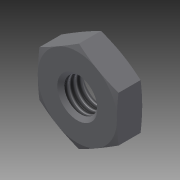
# Autodesk Inventor part: D-5288
Saved by Autodesk Inventor 2014 (Build 180170000, 170)
## iProperties
Category: PARTsolutions
Company: BIMBA
Created: 2014-01-19
Part Number: D-5288
Material: Generic
Catalog Web Link: www.cadenas.de
Description: Mounting Nut for Original Line Cylinders-
Vendor: BIMBA
Document SubType Name: Standard Catalog Part
Designer: Michael
Manufacturer: BIMBA
Density: 1 g/cm^3
Appearance: RGB(191.25000000000000,191.25000000000000,191.25000000000000)
PSOL_IDENT_0: {$CADENAS_DATA\23d-libs\bimba\bimba\bimba_imperial\bimba_full_line\original_line_cylinders\accessori
PSOL_IDENT_1: es\mounting_nut.prj},192 {VTYP=3D},{NB=D-5288},{LINA=D-5288},{NN=Mounting Nut for Original Line Cyli
PSOL_IDENT_2: nders},{DATE=11.06.2012 07:31:25},{GEOMDATE=10.11.2011 00:00:00},{VERSION=},{LINEID=210},{LINESUBID=
PSOL_IDENT_3: -1},{WBVAR=MAT}  {NB=D-5288},{LINA=D-5288},{KT=DUMMY},{PN=D-5288},{PN1=D-5288},{C=#10-32},{TH=UNF},{
PSOL_IDENT_4: MAT=},{MAT1='','Zinc-Plated Carbon Steel', '-SS', 'Stainless Steel'},{A=0.38},{A1=0.37500000},{B=0.1
PSOL_IDENT_5: 2},{B1=0.12000000},{NDM=0.19000000},{PITCH=0.0313},{DIA=-},{DIA2=-},{DIA3=-},{DIA1=0},{DIA4=0.000000
PSOL_IDENT_6: 00},{DIA5=0.00000000},{T=-},{T2=-},{T3=-},{T1=0},{T4=0.00000000},{T5=0.00000000},{COLOR=0.75,0.75,0.
PSOL_IDENT_7: 75,0.00},{TT=0.05000000},{TO=0.20000000},{PRA=1}
CNS_NN: Mounting Nut for Original Line Cylinders
CNS_NB: D-5288
CNS_NBSYN: $PN.
CNS_LINA: D-5288
CNS_PN: D-5288
CNS_PN1: D-5288
CNS_C: #10-32
CNS_TH: UNF
CNS_MAT: Zinc-Plated Carbon Steel
CNS_MAT1: '','Zinc-Plated Carbon Steel', '-SS', 'Stainless Steel'
CNS_A: 0.38
CNS_A1: 0.37500000
CNS_B: 0.12
CNS_B1: 0.12000000
CNS_NDM: 0.19000000
CNS_PITCH: 0.0313
CNS_DIA: -
CNS_DIA2: -
CNS_DIA3: -
CNS_DIA1: 0.000
CNS_DIA4: 0.00000000
CNS_DIA5: 0.00000000
CNS_T: -
CNS_T2: -
CNS_T3: -
CNS_T1: 0.000
CNS_T4: 0.00000000
CNS_T5: 0.00000000
CNS_COLOR: 0.75,0.75,0.75,0.00
CNS_TT: 0.05000000
CNS_TO: 0.20000000
CNS_PRA: 1
SUPPLIER: BIMBA
ARTICLENO: D-5288
BOMINFO: D-5288
CREATOR: CADENAS GmbH
Title: D-5288
Author: Cadenas PARTsolutions
Autodesk Inventor part; units mm, degrees
sketch "Sketch_8" plane through (0, 0, 0) normal (1, 0, 0) x (0, 1, 0)
  line L0 (0, -3.048) -> (0, 0)
  line L1 (0, 0) -> (4.7625, 0)
  line L2 (4.7625, 0) -> (5.715, -0.2552)
  line L3 (5.715, -0.2552) -> (5.715, -2.7928)
  line L4 (5.715, -2.7928) -> (4.7625, -3.048)
  line L5 (4.7625, -3.048) -> (0, -3.048)
  line L6 (0, -3.048) -> (0, 0)
  constraints: 14 end point
sketch "Sketch_10" plane through (0, 0, 0) normal (0, 0, 1) x (1, 0, 0)
  line L0 (-9.525, 9.525) -> (-9.525, -9.525)
  line L1 (-9.525, -9.525) -> (9.525, -9.525)
  line L2 (9.525, -9.525) -> (9.525, 9.525)
  line L3 (9.525, 9.525) -> (-9.525, 9.525)
  line L4 (-4.7625, 2.7496) -> (-4.7625, -2.7496)
  line L5 (-4.7625, -2.7496) -> (0, -5.4993)
  line L6 (0, -5.4993) -> (4.7625, -2.7496)
  line L7 (4.7625, -2.7496) -> (4.7625, 2.7496)
  line L8 (4.7625, 2.7496) -> (0, 5.4993)
  line L9 (0, 5.4993) -> (-4.7625, 2.7496)
  constraints: 20 end point
revolve "Revolution1" add sketch "Sketch_8" angle 360 about axis through (0, 0, -3.048) along (0, 0, -1)
extrude "Extrusion1" cut sketch "Sketch_10" against normal blind 3.048
sketch "Sketch_11" plane through (0, 0, 0) normal (1, 0, 0) x (0, 1, 0)
  line L0 (0, -3.048) -> (0, 0)
  line L1 (0, 0) -> (2.413, 0)
  line L2 (2.413, 0) -> (1.9837, -0.4293)
  line L3 (1.9837, -0.4293) -> (1.9837, -2.6187)
  line L4 (1.9837, -2.6187) -> (2.413, -3.048)
  line L5 (2.413, -3.048) -> (0, -3.048)
  line L6 (0, -3.048) -> (0, 0)
  constraints: 14 end point
revolve "Revolution2" cut sketch "Sketch_11" angle 360 about axis through (0, 0, -3.048) along (0, 0, -1)
thread "Thread1" size "10-32 UNF" class "2B" standard "ANSI Unified Screw Threads" full length
ref_plane "NUT_XY" through (0, 0, 0) normal (0, 0, 1) x (1, 0, 0)
ref_plane "NUT_YZ" through (0, 0, 0) normal (1, 0, 0) x (0, 1, 0)
ref_plane "NUT_ZX" through (0, 0, 0) normal (0, 1, 0) x (0, 0, 1)
ref_plane "a1_XY" through (-4.7625, 4.7625, 0) normal (0, 0, 1) x (1, 0, 0)
ref_plane "a1_YZ" through (-4.7625, 4.7625, 0) normal (1, 0, 0) x (0, 1, 0)
ref_plane "a1_ZX" through (-4.7625, 4.7625, 0) normal (0, 1, 0) x (0, 0, 1)
ref_plane "a2_XY" through (4.7625, 4.7625, 0) normal (0, 0, 1) x (1, 0, 0)
ref_plane "a2_YZ" through (4.7625, 4.7625, 0) normal (1, 0, 0) x (0, 1, 0)
ref_plane "a2_ZX" through (4.7625, 4.7625, 0) normal (0, 1, 0) x (0, 0, 1)
ref_plane "b1_XY" through (0, 4.7625, 0) normal (1, 0, 0) x (0, 0, -1)
ref_plane "b1_YZ" through (0, 4.7625, 0) normal (0, 0, -1) x (0, 1, 0)
ref_plane "b1_ZX" through (0, 4.7625, 0) normal (0, 1, 0) x (1, 0, 0)
ref_plane "b2_XY" through (0, 4.7625, -3.048) normal (1, 0, 0) x (0, 0, -1)
ref_plane "b2_YZ" through (0, 4.7625, -3.048) normal (0, 0, -1) x (0, 1, 0)
ref_plane "b2_ZX" through (0, 4.7625, -3.048) normal (0, 1, 0) x (1, 0, 0)
ref_plane "e_XY" through (0, 0, -3.048) normal (1, 0, 0) x (0, 0, -1)
ref_plane "e_YZ" through (0, 0, -3.048) normal (0, 0, -1) x (0, 1, 0)
ref_plane "e_ZX" through (0, 0, -3.048) normal (0, 1, 0) x (1, 0, 0)
ref_plane "ol1_XY" through (0, 0, -4.7625) normal (0, 1, 0) x (1, 0, 0)
ref_plane "ol1_YZ" through (0, 0, -4.7625) normal (1, 0, 0) x (0, 0, -1)
ref_plane "ol1_ZX" through (0, 0, -4.7625) normal (0, 0, -1) x (0, 1, 0)
ref_plane "ol2_XY" through (3.048, 0, -4.7625) normal (0, 1, 0) x (1, 0, 0)
ref_plane "ol2_YZ" through (3.048, 0, -4.7625) normal (1, 0, 0) x (0, 0, -1)
ref_plane "ol2_ZX" through (3.048, 0, -4.7625) normal (0, 0, -1) x (0, 1, 0)
ref_plane "th1_XY" through (0, 2.413, -3.048) normal (1, 0, 0) x (0, 0, -1)
ref_plane "th1_YZ" through (0, 2.413, -3.048) normal (0, 0, -1) x (0, 1, 0)
ref_plane "th1_ZX" through (0, 2.413, -3.048) normal (0, 1, 0) x (1, 0, 0)
ref_plane "th2_XY" through (0, -2.413, -3.048) normal (1, 0, 0) x (0, 0, -1)
ref_plane "th2_YZ" through (0, -2.413, -3.048) normal (0, 0, -1) x (0, 1, 0)
ref_plane "th2_ZX" through (0, -2.413, -3.048) normal (0, 1, 0) x (1, 0, 0)
body "Solid1"
